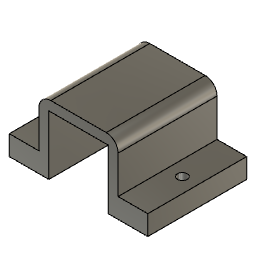
EncaixeMotor v1 (Autodesk Fusion 360 design; units mm, degrees)
Autodesk Fusion 360 part; units mm, degrees
sketch "Esboço1" plane through (0, 0, 0) normal (0, 1, 0) x (1, 0, 0)
  line L0 (-74.1987, -2.4172) -> (-64.1987, -2.4172)
  line L1 (-64.1987, -2.4172) -> (-64.1987, -17.4172)
  line L2 (-64.1987, -17.4172) -> (-49.1987, -17.4172)
  line L3 (-49.1987, -17.4172) -> (-49.1987, -1)
  line L4 (-49.1987, -1) -> (-49.1987, -2.4172)
  line L5 (-49.1987, -2.4172) -> (-39.1987, -2.4172)
  line L6 (-39.1987, -2.4172) -> (-39.1987, -7.4172)
  line L7 (-74.1987, -2.4172) -> (-74.1987, -7.4172)
  line L8 (-74.1987, -7.4172) -> (-66.6987, -7.4172)
  line L9 (-66.6987, -7.4172) -> (-66.6987, -16.9172)
  line L10 (-39.1987, -7.4172) -> (-46.6987, -7.4172)
  line L11 (-46.6987, -7.4172) -> (-46.6987, -16.9172)
  line L12 (-63.6987, -19.9172) -> (-49.6987, -19.9172)
  arc A0 (-66.6987, -16.9172) -> (-63.6987, -19.9172) centre (-63.6987, -16.9172) ccw
  arc A1 (-49.6987, -19.9172) -> (-46.6987, -16.9172) centre (-49.6987, -16.9172) ccw
  point P0 (-66.6987, -19.9172)
  point P1 (-46.6987, -19.9172)
  dimension "d1" = 10
  dimension "d2" = 15
  dimension "d3" = 15
  dimension "d4" = 10
  dimension "d5" = 5
  dimension "d6" = 5
  dimension "d7" = 7.5
  dimension "d8" = 12.5
  dimension "d9" = 7.5
  dimension "d10" = 12.5
  dimension "d11" = 3
  constraint horizontal L0
  constraint perpendicular L0 L1
  constraint perpendicular L1 L2
  constraint perpendicular L2 L3
  constraint perpendicular L2 L4
  constraint perpendicular L4 L5
  constraint perpendicular L5 L6
  constraint perpendicular L0 L7
  constraint perpendicular L7 L8
  constraint perpendicular L8 L9
  constraint perpendicular L6 L10
  constraint perpendicular L10 L11
  constraint perpendicular L11 L12
  constraint coincident P0 L9
  constraint coincident P0 L12
  constraint tangent L9 A0
  constraint tangent L12 A0
  constraint coincident P1 L11
  constraint coincident P1 L12
  constraint tangent L11 A1
  constraint tangent L12 A1
  constraint equal A0 A1
  measures "d1" distance of L0.start L0.end
  measures "d2" distance of L0.end L1.end
  measures "d3" distance of L1.end L2.end
  measures "d4" distance of L4.end L5.end
  measures "d5" distance of L5.end L6.end
  measures "d6" distance of L0.start L7.end
  measures "d7" distance of L7.end L8.end
  measures "d8" distance of L8.end P0
  measures "d9" distance of L6.end L10.end
  measures "d10" distance of L10.end P1
  measures "d11" radius of A0
extrude "Extrusão1" add sketch "Esboço1" along normal blind 25
sketch "Esboço2" plane through (0, 0, 0) normal (0, 0, 1) x (1, 0, 0)
hole "Furo1" at (-70.4487, 12.5, 7.4172) direction (0, 0, -1) diameter 2.5 depth 9 tip angle 118
hole "Furo2" at (-42.9487, 12.5, 7.4172) direction (0, 0, -1) diameter 2.5 depth 9 tip angle 118
